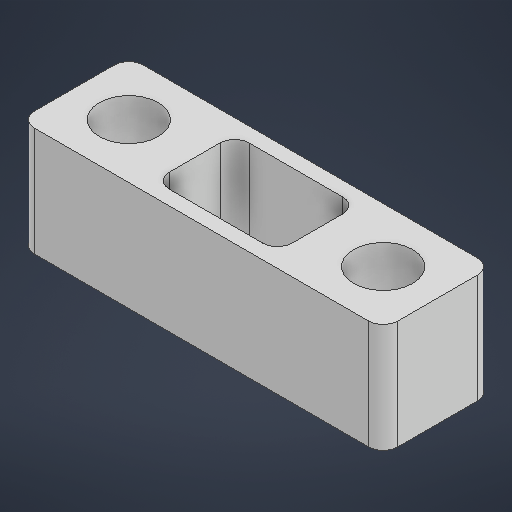
# Autodesk Inventor part: Support_Seperator
Saved by Autodesk Inventor 2026.2 (Build 302298000, 298)
## iProperties
Created: 2025-12-17
Part Number: Support_Seperator
Material: Generic
Document SubType Name: Modeling
Designer: Cobble
Density: 1 g/cm^3
Appearance: Default
Author: Cobble
Autodesk Inventor part; units mm, degrees
ref_plane "YZ Plane" through (0, 0, 0) normal (1, 0, 0) x (0, 1, 0)
ref_plane "XZ Plane" through (0, 0, 0) normal (0, 1, 0) x (-1, 0, 0)
ref_plane "XY Plane" through (0, 0, 0) normal (0, 0, 1) x (1, 0, 0)
sketch "Sketch1" plane through (0, 0, 0) normal (0, 0, 1) x (1, 0, 0)
  line L0 (0, 0) -> (50, 0)
  line L1 (50, 0) -> (50, -15)
  line L2 (50, -15) -> (0, -15)
  line L3 (0, -15) -> (0, 0)
  line L4 (0, 0) -> (15, -15)
  line L5 (0, 0) -> (21.2132, 0) construction
  circle A0 centre (7.5, -7.5) radius 4.05
  line L6 (50, 0) -> (35, -15)
  circle A1 centre (42.5, -7.5) radius 4.05
  line L7 (11.55, -7.5) -> (16.55, -7.5)
  line L8 (25, -15) -> (25, -13)
  line L9 (25, 0) -> (25, -2)
  line L10 (33.45, -13) -> (16.55, -13)
  line L11 (16.55, -13) -> (16.55, -2)
  line L12 (16.55, -2) -> (33.45, -2)
  line L13 (33.45, -2) -> (33.45, -13)
  line L14 (33.45, -13) -> (16.55, -2) construction
  line L15 (16.55, -13) -> (33.45, -2) construction
  point P0 (25, -7.5)
  dimension "d3" = 8.1
  dimension "d0" = 50
  dimension "d1" = 15
  dimension "d2" = 45
  dimension "d4" = 8.1
  dimension "d5" = 45
  dimension "d9" = 5
  dimension "d10" = 2
  dimension "d11" = 2
  constraints: 32 end point, 6 midpoint, 4 horizontal, 4 parallel, 2 perpendicular, 2 point on line, 2 vertical, 1 centre point, 1 equal length, 1 horizontal alignment, 2 other
  measures "d0" distance of L1.end L2.end
  measures "d1" distance of L0.end L1.end
  measures "d2" angle of L4 L5
  measures "d4" diameter of A1
  measures "d5" angle of L0 L6
  measures "d9" distance of L7.start L7.end
  measures "d10" distance of L8.start L8.end
  measures "d11" distance of L9.start L9.end
extrude "Extrusion1" add sketch "Sketch1" along normal blind 15 contours L4 A0 L2 L3 | L0 L9 L12 L11 L7 A0 L4 | L0 L6 A1 L2 L8 L10 L13 L12 L9 | L1 L2 L6 A1 | L4 A0 L7 L11 L10 L8 L2
fillet "Fillet1" radius 2 8 edges at (50, 0, 7.5) (50, -15, 7.5) (0, 0, 7.5) (0, -15, 7.5) (16.55, -13, 7.5) (16.55, -2, 7.5) (33.45, -2, 7.5) (33.45, -13, 7.5)
body "Solid1"
